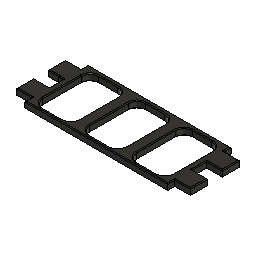
Cadran Numere (Autodesk Fusion 360 design; units mm, degrees)
part number: 2026-05-27-02-16-51-186
Autodesk Fusion 360 part; units mm, degrees
sketch "Sketch1" plane through (0, 0, 0) normal (0, 0, 1) x (1, 0, 0)
  line L0 (40, 20) -> (128, 20)
  line L1 (40, 20) -> (40, 24)
  line L2 (40, 24) -> (34, 24)
  line L3 (34, 24) -> (34, 34)
  line L4 (34, 34) -> (40, 34)
  line L5 (40, 34) -> (40, 42.3)
  line L6 (40, 42.3) -> (34, 42.3)
  line L7 (34, 42.3) -> (34, 52.3)
  line L8 (34, 52.3) -> (40, 52.3)
  line L9 (40, 52.3) -> (40, 56.3)
  line L10 (40, 56.3) -> (128, 56.3)
  line L11 (128, 56.3) -> (128, 52.3)
  line L12 (128, 52.3) -> (134, 52.3)
  line L13 (134, 52.3) -> (134, 42.3)
  line L14 (134, 42.3) -> (128, 42.3)
  line L15 (128, 42.3) -> (128, 34)
  line L16 (128, 34) -> (134, 34)
  line L17 (134, 34) -> (134, 24)
  line L18 (134, 24) -> (128, 24)
  line L19 (128, 24) -> (128, 20)
  line L20 (51.5, 53.8) -> (62.5, 53.8)
  line L21 (67.5, 48.8) -> (67.5, 26.8)
  line L22 (62.5, 21.8) -> (51.5, 21.8)
  line L23 (46.5, 26.8) -> (46.5, 48.8)
  line L24 (78.5, 53.8) -> (89.5, 53.8)
  line L25 (94.5, 48.8) -> (94.5, 26.8)
  line L26 (89.5, 21.8) -> (78.5, 21.8)
  line L27 (73.5, 26.8) -> (73.5, 48.8)
  line L28 (105.5, 53.8) -> (116.5, 53.8)
  line L29 (121.5, 48.8) -> (121.5, 26.8)
  line L30 (116.5, 21.8) -> (105.5, 21.8)
  line L31 (100.5, 26.8) -> (100.5, 48.8)
  arc A0 (51.5, 53.8) -> (46.5, 48.8) centre (51.5, 48.8) ccw
  arc A1 (67.5, 48.8) -> (62.5, 53.8) centre (62.5, 48.8) ccw
  arc A2 (46.5, 26.8) -> (51.5, 21.8) centre (51.5, 26.8) ccw
  arc A3 (62.5, 21.8) -> (67.5, 26.8) centre (62.5, 26.8) ccw
  arc A4 (78.5, 53.8) -> (73.5, 48.8) centre (78.5, 48.8) ccw
  arc A5 (73.5, 26.8) -> (78.5, 21.8) centre (78.5, 26.8) ccw
  arc A6 (89.5, 21.8) -> (94.5, 26.8) centre (89.5, 26.8) ccw
  arc A7 (94.5, 48.8) -> (89.5, 53.8) centre (89.5, 48.8) ccw
  arc A8 (105.5, 53.8) -> (100.5, 48.8) centre (105.5, 48.8) ccw
  arc A9 (121.5, 48.8) -> (116.5, 53.8) centre (116.5, 48.8) ccw
  arc A10 (100.5, 26.8) -> (105.5, 21.8) centre (105.5, 26.8) ccw
  arc A11 (116.5, 21.8) -> (121.5, 26.8) centre (116.5, 26.8) ccw
  point P0 (46.5, 53.8)
  point P1 (67.5, 53.8)
  point P2 (46.5, 21.8)
  point P3 (73.5, 53.8)
  point P4 (94.5, 53.8)
  point P5 (73.5, 21.8)
  point P6 (100.5, 53.8)
  point P7 (121.5, 53.8)
  point P8 (100.5, 21.8)
  dimension "d1" = 88
  dimension "d2" = 4
  dimension "d3" = 6
  dimension "d4" = 10
  dimension "d5" = 6
  dimension "d6" = 8.3
  dimension "d7" = 6
  dimension "d8" = 10
  dimension "d9" = 6
  dimension "d10" = 4
  dimension "d11" = 88
  dimension "d12" = 4
  dimension "d13" = 6
  dimension "d14" = 10
  dimension "d15" = 6
  dimension "d16" = 8.3
  dimension "d17" = 6
  dimension "d18" = 10
  dimension "d21" = 21
  dimension "d22" = 32
  dimension "d23" = 6
  dimension "d24" = 21
  dimension "d25" = 32
  dimension "d26" = 6
  dimension "d27" = 21
  dimension "d28" = 32
  dimension "d29" = 5
  constraint horizontal L0
  constraint perpendicular L0 L1
  constraint perpendicular L1 L2
  constraint perpendicular L2 L3
  constraint perpendicular L3 L4
  constraint perpendicular L4 L5
  constraint perpendicular L5 L6
  constraint perpendicular L6 L7
  constraint perpendicular L7 L8
  constraint perpendicular L8 L9
  constraint perpendicular L9 L10
  constraint perpendicular L10 L11
  constraint perpendicular L11 L12
  constraint perpendicular L12 L13
  constraint perpendicular L13 L14
  constraint perpendicular L14 L15
  constraint perpendicular L15 L16
  constraint perpendicular L16 L17
  constraint perpendicular L17 L18
  constraint horizontal L20
  constraint vertical L21
  constraint horizontal L22
  constraint vertical L23
  constraint horizontal L24
  constraint vertical L25
  constraint horizontal L26
  constraint vertical L27
  constraint horizontal L28
  constraint vertical L29
  constraint horizontal L30
  constraint vertical L31
  constraint coincident P0 L20
  constraint coincident P0 L23
  constraint tangent L20 A0
  constraint tangent L23 A0
  constraint coincident P1 L20
  constraint coincident P1 L21
  constraint tangent L20 A1
  constraint tangent L21 A1
  constraint equal A0 A1
  constraint coincident P2 L23
  constraint coincident P2 L22
  constraint tangent L23 A2
  constraint tangent L22 A2
  constraint equal A0 A2
  constraint tangent L21 A3
  constraint tangent L22 A3
  constraint equal A0 A3
  constraint coincident P3 L24
  constraint coincident P3 L27
  constraint tangent L24 A4
  constraint tangent L27 A4
  constraint equal A0 A4
  constraint coincident P5 L27
  constraint coincident P5 L26
  constraint tangent L27 A5
  constraint tangent L26 A5
  constraint equal A0 A5
  constraint tangent L26 A6
  constraint tangent L25 A6
  constraint equal A0 A6
  constraint coincident P4 L25
  constraint coincident P4 L24
  constraint tangent L25 A7
  constraint tangent L24 A7
  constraint equal A0 A7
  constraint coincident P6 L28
  constraint coincident P6 L31
  constraint tangent L28 A8
  constraint tangent L31 A8
  constraint equal A0 A8
  constraint coincident P7 L28
  constraint coincident P7 L29
  constraint tangent L28 A9
  constraint tangent L29 A9
  constraint equal A0 A9
  constraint coincident P8 L31
  constraint coincident P8 L30
  constraint tangent L31 A10
  constraint tangent L30 A10
  constraint equal A0 A10
  constraint tangent L29 A11
  constraint tangent L30 A11
  constraint equal A0 A11
  measures "d1" distance of L0.start L0.end
  measures "d2" distance of L0.start L1.end
  measures "d3" distance of L1.end L2.end
  measures "d4" distance of L2.end L3.end
  measures "d5" distance of L3.end L4.end
  measures "d6" distance of L4.end L5.end
  measures "d7" distance of L5.end L6.end
  measures "d8" distance of L6.end L7.end
  measures "d9" distance of L7.end L8.end
  measures "d10" distance of L8.end L9.end
  measures "d11" distance of L9.end L10.end
  measures "d12" distance of L10.end L11.end
  measures "d13" distance of L11.end L12.end
  measures "d14" distance of L12.end L13.end
  measures "d15" distance of L13.end L14.end
  measures "d16" distance of L14.end L15.end
  measures "d17" distance of L15.end L16.end
  measures "d18" distance of L16.end L17.end
  measures "d21" distance of P0 P1
  measures "d22" distance of P0 P2
  measures "d23" distance of P1 P3
  measures "d24" distance of P3 P4
  measures "d25" distance of P3 P5
  measures "d26" distance of P4 P6
  measures "d27" distance of P6 P7
  measures "d28" distance of P6 P8
  measures "d29" radius of A0
extrude "Extrude1" add sketch "Sketch1" along normal blind 4
sketch "Sketch2" plane through (0, 0, 4) normal (0, 0, 1) x (-1, 0, 0)
  arc A0 (-100.5, -26.8) -> (-105.5, -21.8) centre (-105.5, -26.8) ccw
  line L0 (-100.5, -26.8) -> (-100.5, -48.8)
  arc A1 (-105.5, -53.8) -> (-100.5, -48.8) centre (-105.5, -48.8) ccw
  line L1 (-105.5, -53.8) -> (-116.5, -53.8)
  arc A2 (-121.5, -48.8) -> (-116.5, -53.8) centre (-116.5, -48.8) ccw
  line L2 (-121.5, -48.8) -> (-121.5, -26.8)
  arc A3 (-116.5, -21.8) -> (-121.5, -26.8) centre (-116.5, -26.8) ccw
  line L3 (-116.5, -21.8) -> (-105.5, -21.8)
  arc A4 (-89.5, -21.8) -> (-94.5, -26.8) centre (-89.5, -26.8) ccw
  line L4 (-89.5, -21.8) -> (-78.5, -21.8)
  arc A5 (-73.5, -26.8) -> (-78.5, -21.8) centre (-78.5, -26.8) ccw
  line L5 (-73.5, -26.8) -> (-73.5, -48.8)
  arc A6 (-78.5, -53.8) -> (-73.5, -48.8) centre (-78.5, -48.8) ccw
  line L6 (-78.5, -53.8) -> (-89.5, -53.8)
  arc A7 (-94.5, -48.8) -> (-89.5, -53.8) centre (-89.5, -48.8) ccw
  line L7 (-94.5, -48.8) -> (-94.5, -26.8)
  arc A8 (-46.5, -26.8) -> (-51.5, -21.8) centre (-51.5, -26.8) ccw
  line L8 (-46.5, -26.8) -> (-46.5, -48.8)
  arc A9 (-51.5, -53.8) -> (-46.5, -48.8) centre (-51.5, -48.8) ccw
  line L9 (-51.5, -53.8) -> (-62.5, -53.8)
  arc A10 (-67.5, -48.8) -> (-62.5, -53.8) centre (-62.5, -48.8) ccw
  line L10 (-67.5, -48.8) -> (-67.5, -26.8)
  arc A11 (-62.5, -21.8) -> (-67.5, -26.8) centre (-62.5, -26.8) ccw
  line L11 (-62.5, -21.8) -> (-51.5, -21.8)
  line L12 (-40, -20) -> (-128, -20)
  line L13 (-128, -20) -> (-128, -24)
  line L14 (-128, -24) -> (-134, -24)
  line L15 (-134, -24) -> (-134, -34)
  line L16 (-134, -34) -> (-128, -34)
  line L17 (-128, -34) -> (-128, -42.3)
  line L18 (-128, -42.3) -> (-134, -42.3)
  line L19 (-134, -42.3) -> (-134, -52.3)
  line L20 (-134, -52.3) -> (-128, -52.3)
  line L21 (-128, -52.3) -> (-128, -56.3)
  line L22 (-128, -56.3) -> (-40, -56.3)
  line L23 (-40, -56.3) -> (-40, -52.3)
  line L24 (-40, -52.3) -> (-34, -52.3)
  line L25 (-34, -52.3) -> (-34, -42.3)
  line L26 (-34, -42.3) -> (-40, -42.3)
  line L27 (-40, -42.3) -> (-40, -34)
  line L28 (-40, -34) -> (-34, -34)
  line L29 (-34, -34) -> (-34, -24)
  line L30 (-34, -24) -> (-40, -24)
  line L31 (-40, -24) -> (-40, -20)
  line L32 (-40, -56.3) -> (-43, -56.3)
  line L33 (-43, -56.3) -> (-43, -20)
  line L34 (-43, -20) -> (-40, -20)
  line L35 (-40, -20) -> (-40, -56.3)
  line L36 (-128, -56.3) -> (-125, -56.3)
  line L37 (-125, -56.3) -> (-125, -20)
  line L38 (-125, -20) -> (-128, -20)
  line L39 (-128, -20) -> (-128, -56.3)
  line L40 (-128, -52.3) -> (-125, -52.3)
  line L41 (-125, -52.3) -> (-125, -42.3)
  line L42 (-125, -42.3) -> (-128, -42.3)
  line L43 (-128, -42.3) -> (-128, -52.3)
  line L44 (-128, -34) -> (-125, -34)
  line L45 (-125, -34) -> (-125, -24)
  line L46 (-125, -24) -> (-128, -24)
  line L47 (-128, -24) -> (-128, -34)
  line L48 (-40, -52.3) -> (-43, -52.3)
  line L49 (-43, -52.3) -> (-43, -42)
  line L50 (-43, -42) -> (-40, -42)
  line L51 (-40, -42) -> (-40, -52.3)
  line L52 (-40, -34) -> (-43, -34)
  line L53 (-43, -34) -> (-43, -24)
  line L54 (-43, -24) -> (-40, -24)
  line L55 (-40, -24) -> (-40, -34)
  line L56 (-40, -42) -> (-43, -42)
  line L57 (-43, -42) -> (-43, -34)
  line L58 (-43, -34) -> (-40, -34)
  line L59 (-40, -34) -> (-40, -42)
  line L60 (-40, -56.3) -> (-43, -56.3)
  line L61 (-43, -56.3) -> (-43, -52.3)
  line L62 (-43, -52.3) -> (-40, -52.3)
  line L63 (-40, -52.3) -> (-40, -56.3)
  line L64 (-40, -24) -> (-43, -24)
  line L65 (-43, -24) -> (-43, -20)
  line L66 (-43, -20) -> (-40, -20)
  line L67 (-40, -20) -> (-40, -24)
  line L68 (-125, -56.3) -> (-128, -56.3)
  line L69 (-128, -56.3) -> (-128, -52.3)
  line L70 (-128, -52.3) -> (-125, -52.3)
  line L71 (-125, -52.3) -> (-125, -56.3)
  line L72 (-125, -42.3) -> (-128, -42.3)
  line L73 (-128, -42.3) -> (-128, -34)
  line L74 (-128, -34) -> (-125, -34)
  line L75 (-125, -34) -> (-125, -42.3)
  line L76 (-125, -24) -> (-128, -24)
  line L77 (-128, -24) -> (-128, -20)
  line L78 (-128, -20) -> (-125, -20)
  line L79 (-125, -20) -> (-125, -24)
  constraint horizontal L32
  constraint vertical L33
  constraint horizontal L34
  constraint vertical L35
  constraint coincident L12 L33.end
  constraint coincident L22.end L23.start
  constraint horizontal L36
  constraint vertical L37
  constraint horizontal L38
  constraint vertical L39
  constraint coincident L12 L37.end
  constraint coincident L21.end L22.start
  constraint horizontal L40
  constraint vertical L41
  constraint horizontal L42
  constraint vertical L43
  constraint coincident L37 L41.end
  constraint coincident L20.end L21.start
  constraint horizontal L44
  constraint vertical L45
  constraint horizontal L46
  constraint vertical L47
  constraint coincident L37 L45.end
  constraint coincident L16.end L17.start
  constraint horizontal L48
  constraint vertical L49
  constraint horizontal L50
  constraint vertical L51
  constraint coincident L33 L49.end
  constraint coincident L23.end L24.start
  constraint horizontal L52
  constraint vertical L53
  constraint horizontal L54
  constraint vertical L55
  constraint coincident L33 L53.end
  constraint coincident L27.end L28.start
  constraint horizontal L56
  constraint vertical L57
  constraint horizontal L58
  constraint vertical L59
  constraint horizontal L60
  constraint vertical L61
  constraint horizontal L62
  constraint vertical L63
  constraint horizontal L64
  constraint vertical L65
  constraint horizontal L66
  constraint vertical L67
  constraint horizontal L68
  constraint vertical L69
  constraint horizontal L70
  constraint vertical L71
  constraint horizontal L72
  constraint vertical L73
  constraint horizontal L74
  constraint vertical L75
  constraint horizontal L76
  constraint vertical L77
  constraint horizontal L78
  constraint vertical L79
extrude "Extrude2" cut sketch "Sketch2" against normal blind 40 contours L12 L31 L33 L34 L35 L54 L64 L65 L66 L67 | L12 L13 L37 L38 L39 L46 L76 L77 L78 L79 | L27 L33 L35 L50 L52 L56 L57 L58 L59 | L17 L37 L39 L42 L44 L72 L73 L74 L75 | L22 L23 L32 L33 L35 L48 L60 L61 L62 L63 | L21 L22 L36 L37 L39 L40 L68 L69 L70 L71
chamfer "Chamfer1" distance 0.5 angle 45 1 faces at (39, 30.6667, 4)
chamfer "Chamfer2" distance 0.5 angle 45 1 faces at (39, 30.6667, 0)
